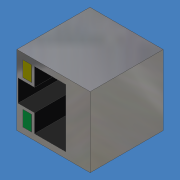
# Autodesk Inventor part: cRIO-FRC CAT5
Saved by Autodesk Inventor 2011 (Build 150239000, 239)
## iProperties
Category: FRC Parts
Manager: Ed Sparks
Company: FirstCadLibrary
Shininess: 64.0
Length Units: 11272
Angle Units: 11279
Time Units: 11290
Mass Units: 11286
Length Display Precision: 3
Angle Display Precision: 2
Compacted: True
Part Number: cRIO-FRC CAT5
Document SubType Name: Modeling
Created: 2008-12-16
Designer: Ed Sparks
Project: FIRST
Catalog Web Link: www.firstcadlibrary.com
Engineer: Ed Sparks
Material: ABS Plastic
Density: 1 g/cm^3
Density: 0.0
Volumn: 0.0
Area: 0.0
PropertySet Name: Model Information
Control State: 0
Master: False
Checked Out: False
Author: Ed Sparks
Keywords: FIRST
Autodesk Inventor part; units mm, degrees
ref_plane "YZ Plane" through (0, 0, 0) normal (1, 0, 0) x (0, 1, 0)
ref_plane "XZ Plane" through (0, 0, 0) normal (0, 1, 0) x (-1, 0, 0)
ref_plane "XY Plane" through (0, 0, 0) normal (0, 0, 1) x (1, 0, 0)
sketch "Sketch1" plane through (0, 0, 0) normal (0, 0, 1) x (1, 0, 0)
  line L0 (-8.4582, 8.1026) -> (8.4582, 8.1026)
  line L1 (8.4582, 8.1026) -> (8.4582, -8.1026)
  line L2 (8.4582, -8.1026) -> (-8.4582, -8.1026)
  line L3 (-8.4582, -8.1026) -> (-8.4582, 8.1026)
  line L4 (0, 0) -> (0, 8.1026) construction
  line L5 (0, 0) -> (0, -8.1026) construction
  line L6 (0, 0) -> (-8.4582, 0) construction
  line L7 (0, 0) -> (8.4582, 0) construction
  dimension "d0" = 16.9164
  dimension "d1" = 16.2052
  constraints: 16 end point, 4 midpoint, 2 collinear, 2 parallel, 1 horizontal, 1 perpendicular, 1 other
  measures "d0" distance of L0.start L0.end
  measures "d1" distance of L2.end L0.start
extrude "Extrusion1" add sketch "Sketch1" along normal mid plane 16.8656
sketch "Sketch2" plane through (0, 0, 8.4328) normal (0, 0, 1) x (1, 0, 0)
  line L0 (8.4582, 8.1026) -> (8.4582, -8.1026) projected
  line L1 (-8.4582, 8.1026) -> (8.4582, 8.1026) projected
  line L2 (-8.4582, -8.1026) -> (-8.4582, 8.1026) projected
  line L3 (8.4582, -8.1026) -> (-8.4582, -8.1026) projected
  line L4 (-8.2042, -2.54) -> (-8.2042, 2.54)
  line L5 (-8.2042, 2.54) -> (-4.3942, 2.54)
  line L6 (-4.3942, 2.54) -> (-4.3942, 6.731)
  line L7 (-4.3942, 6.731) -> (2.8702, 6.731)
  line L8 (2.8702, 6.731) -> (2.8702, -6.731)
  line L9 (2.8702, -6.731) -> (-4.3942, -6.731)
  line L10 (-4.3942, -6.731) -> (-4.3942, -2.54)
  line L11 (-4.3942, -2.54) -> (-8.2042, -2.54)
  line L12 (0, 8.1026) -> (0, -8.1026) construction
  line L13 (-8.4582, 0) -> (8.4582, 0) construction
  dimension "d4" = 13.462
  dimension "d5" = 0.254
  dimension "d6" = 3.81
  dimension "d7" = 5.08
  dimension "d8" = 5.588
  constraints: 20 end point, 4 horizontal, 4 midpoint, 4 vertical, 3 equal length, 2 other
  measures "d4" distance of L7.end L8.end
  measures "d5" distance between parallel lines of L2 L4
  measures "d6" distance of L4.end L5.end
  measures "d7" distance between parallel lines of L11 L5
  measures "d8" distance between parallel lines of L8 L0
extrude "Extrusion2" cut sketch "Sketch2" against normal blind 10.16 contours L4 L5 L6 L7 L8 L9 L10 L11
sketch "Sketch3" plane through (0, 0, 8.4328) normal (0, 0, 1) x (1, 0, 0)
  line L0 (-8.2042, 2.54) -> (-4.3942, 2.54) projected
  line L1 (-4.3942, 2.54) -> (-4.3942, 6.731) projected
  line L2 (-4.3942, 6.731) -> (2.8702, 6.731) projected
  line L3 (-7.0612, 6.731) -> (-5.0292, 6.731)
  line L4 (-5.0292, 6.731) -> (-5.0292, 3.175)
  line L5 (-5.0292, 3.175) -> (-7.0612, 3.175)
  line L6 (-7.0612, 3.175) -> (-7.0612, 6.731)
  dimension "d11" = 0.635
  dimension "d12" = 0.635
  dimension "d13" = 2.032
  constraints: 8 end point, 2 parallel, 1 collinear, 1 horizontal, 1 perpendicular
  measures "d11" distance between parallel lines of L4 L1
  measures "d12" distance between parallel lines of L0 L5
  measures "d13" distance between parallel lines of L6 L4
extrude "Extrusion3" add sketch "Sketch3" along normal blind 0.0254
mirror "Mirror1" about plane through (0, 0, 0) normal (0, 1, 0) of "Extrusion3"
body "Solid1"
